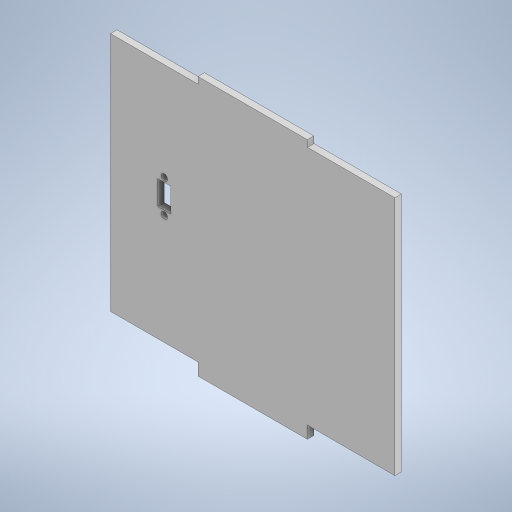
# Autodesk Inventor part: BackWallV2
Saved by Autodesk Inventor 2023 (Build 270158000, 158)
## iProperties
Created: 2022-10-06
Part Number: BackWallV2
Material: Generic
Document SubType Name: Modeling
Designer: digge
Density: 1 g/cm^3
Appearance: Default
Author: digge
Autodesk Inventor part; units mm, degrees
ref_plane "YZ Plane" through (0, 0, 0) normal (1, 0, 0) x (0, 1, 0)
ref_plane "XZ Plane" through (0, 0, 0) normal (0, 1, 0) x (-1, 0, 0)
ref_plane "XY Plane" through (0, 0, 0) normal (0, 0, 1) x (1, 0, 0)
sketch "Sketch1" plane through (0, 0, 0) normal (0, 0, 1) x (1, 0, 0)
  line L0 (-70.131, 85.6788) -> (-70.131, -24.3212)
  line L1 (-70.131, -24.3212) -> (-30.131, -24.3212)
  line L2 (-30.131, -24.3212) -> (-30.131, -29.9212)
  line L3 (-30.131, -29.9212) -> (19.869, -29.9212)
  line L4 (19.869, -29.9212) -> (19.869, -24.3212)
  line L5 (19.869, -24.3212) -> (59.869, -24.3212)
  line L6 (59.869, -24.3212) -> (59.869, 85.6788)
  line L7 (59.869, 85.6788) -> (19.869, 85.6788)
  line L8 (19.869, 85.6788) -> (19.869, 88.6788)
  line L9 (19.869, 88.6788) -> (-30.131, 88.6788)
  line L10 (-30.131, 88.6788) -> (-30.131, 85.6788)
  line L11 (-30.131, 85.6788) -> (-70.131, 85.6788)
  line L12 (-5.131, 88.6788) -> (-5.131, -29.9212) construction
  line L13 (-48.5521, 39.0524) -> (-48.5521, 28.0524)
  line L14 (-48.5521, 28.0524) -> (-42.5521, 28.0524)
  line L15 (-42.5521, 28.0524) -> (-42.5521, 39.0524)
  line L16 (-42.5521, 39.0524) -> (-48.5521, 39.0524)
  circle A0 centre (-45.5521, 41.0524) radius 1.5
  circle A1 centre (-45.5521, 26.0524) radius 1.5
  line L17 (-45.5521, 26.0524) -> (-45.5521, 41.0524) construction
  point P0 (0, 0)
  dimension "d0" = 130
  dimension "d1" = 110
  dimension "d2" = 50
  dimension "d3" = 50
  dimension "d4" = 11
  dimension "d5" = 6
  dimension "d6" = 3
  dimension "d7" = 2
  dimension "d8" = 3
  dimension "d9" = 2
  dimension "d12" = 3
  dimension "d13" = 5.6
  constraints: 36 end point, 12 perpendicular, 3 point on line, 3 vertical, 2 centre point, 2 midpoint, 1 horizontal, 2 other
  measures "d0" distance between parallel lines of L6 L0
  measures "d1" distance of L0.start L0.end
  measures "d2" distance of L8.end L9.end
  measures "d3" distance of L2.end L3.end
  measures "d4" distance of L14.end L15.end
  measures "d5" distance of L15.end L13.start
  measures "d6" diameter of A0
  measures "d7" distance from line of L16 L17.end
  measures "d8" diameter of A1
  measures "d9" distance from line of L14 L17.start
  measures "d12" distance of L7.end L8.end
  measures "d13" distance between parallel lines of L5 L3
extrude "Extrusion1" add sketch "Sketch1" along normal blind 3
body "Solid1"
